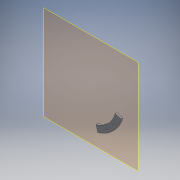
# Autodesk Inventor part: PartBallCupAlignment
Saved by Autodesk Inventor 2016 (Build 200138000, 138)
## iProperties
Created: 2018-01-13
Part Number: PartBallCupAlignment
Material: Generic
Document SubType Name: Modeling
Designer: harveylab
Density: 1 g/cm^3
Appearance: Default
Author: harveylab
Autodesk Inventor part; units mm, degrees
ref_plane "YZ Plane" through (0, 0, 0) normal (1, 0, 0) x (0, 1, 0)
ref_plane "XZ Plane" through (0, 0, 0) normal (0, 1, 0) x (-1, 0, 0)
ref_plane "XY Plane" through (0, 0, 0) normal (0, 0, 1) x (1, 0, 0)
ref_plane "Work Plane1" through (0, 0, 0) normal (0, 0, 1) x (1, 0, 0)
sketch "Sketch1" plane through (0, 0, 0) normal (0, 0, 1) x (1, 0, 0)
  line L0 (0, 0) -> (-152.4, 0)
  circle A0 centre (-38.1, -165.1) radius 2.8067 construction
  line L1 (-60.3956, -177.0525) -> (-38.9279, -182.8048)
  line L2 (-127.7475, -244.4044) -> (-121.9952, -265.8721)
  arc A1 (-127.7475, -244.4044) -> (-60.3956, -177.0525) centre (-152.4, -152.4) ccw
  arc A2 (-121.9952, -265.8721) -> (-38.9279, -182.8048) centre (-152.4, -152.4) ccw
  line L3 (0, 0) -> (-63.5, 0)
  line L4 (-63.5, 0) -> (-63.5, -215.9) construction
  line L5 (-63.5, -215.9) -> (-88.9, -215.9) construction
  line L6 (-88.9, -215.9) -> (-88.9, -241.3) construction
  circle A3 centre (-63.5, -215.9) radius 3.302
  circle A4 centre (-88.9, -241.3) radius 3.302
  dimension "d0" = 152.4
  dimension "d8" = 63.5
  dimension "d9" = 215.9
  dimension "d10" = 25.4
  dimension "d11" = 25.4
  dimension "d12" = 6.604
  dimension "d13" = 6.604
  constraints: 14 end point, 4 centre point, 4 point on circle, 3 coincident, 3 perpendicular, 1 horizontal, 1 point on line
  measures "d0" distance of L0.start L0.end
  measures "d8" distance of L0.start L3.end
  measures "d9" distance of L3.end L4.end
  measures "d10" distance of L4.end L5.end
  measures "d11" distance of L5.end L6.end
  measures "d12" diameter of A3
  measures "d13" diameter of A4
extrude "Extrusion1" add sketch "Sketch1" along normal blind 6.35
body "Solid1"
